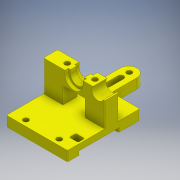
# Autodesk Inventor part: Extruder Mount
Saved by Autodesk Inventor 2016 (Build 200138000, 138)
## iProperties
Created: 2016-03-27
Part Number: Extruder Mount
Material: ABS Plastic
Document SubType Name: Modeling
Designer: Scott
Mass: 47.0424 g
Surface Area: 151.913 cm^2
Volume: 44.3796 cm^3
Density: 1.06 g/cm^3
Appearance: Smooth - Yellow
Author: Scott
Autodesk Inventor part; units mm, degrees
ref_plane "YZ Plane" through (0, 0, 0) normal (1, 0, 0) x (0, 1, 0)
ref_plane "XZ Plane" through (0, 0, 0) normal (0, 1, 0) x (-1, 0, 0)
sketch "Sketch1" plane through (0, 0, 0) normal (0, 0, 1) x (1, 0, 0)
  line L0 (0, 0) -> (85, 0)
  line L1 (85, 0) -> (85, 83.5)
  line L2 (85, 83.5) -> (0, 83.5)
  line L3 (0, 83.5) -> (0, 0)
  dimension "d0" = 85
  dimension "d1" = 83.5
  constraints: 8 end point, 2 parallel, 1 horizontal, 1 perpendicular
  measures "d0" distance of L1.end L2.end
  measures "d1" distance of L0.end L1.end
extrude "Extrusion1" add sketch "Sketch1" along normal blind 5
sketch "Sketch10" plane through (0, 0, 5) normal (0, 0, 1) x (1, 0, 0)
  line L0 (85, 0) -> (85, 83.5) projected
  line L1 (85, 83.5) -> (0, 83.5) projected
  line L2 (0, 83.5) -> (0, 0) projected
  circle A0 centre (15.5, 75) radius 2.25 projected
  circle A1 centre (15.5, 75) radius 4
  circle A2 centre (33.5, 75) radius 4
  circle A3 centre (51.5, 75) radius 4
  circle A4 centre (69.5, 75) radius 4
  circle A5 centre (33.5, 51) radius 2.25 projected
  line L3 (0, 0) -> (85, 0) projected
  circle A6 centre (33.5, 30) radius 4
  circle A7 centre (51.5, 30) radius 4
  circle A8 centre (33.5, 6) radius 4
  circle A9 centre (51.5, 6) radius 4
  line L4 (85, 0) -> (85, 83.5) projected
  line L5 (85, 83.5) -> (0, 83.5) projected
  line L6 (0, 83.5) -> (0, 0) projected
  line L7 (0, 0) -> (85, 0) projected
  circle A10 centre (15.5, 51) radius 2.25 projected
  circle A11 centre (15.5, 51) radius 4
  circle A12 centre (33.5, 51) radius 4
  circle A13 centre (51.5, 51) radius 4
  circle A14 centre (69.5, 51) radius 4
  circle A15 centre (37.75, 40.5) radius 1.5 projected
  circle A16 centre (47.25, 40.5) radius 1.5 projected
  circle A17 centre (37.75, 40.5) radius 2.75
  circle A18 centre (47.25, 40.5) radius 2.75
  dimension "d73" = 8
  dimension "d152" = 5.5
  constraints: 14 centre point, 12 equal radius, 5 coincident
  measures "d73" diameter of A1
  measures "d152" diameter of A17
extrude "Extrusion21" add sketch "Sketch10" along normal blind 4 contours L3 L2 L1 L0 | A0 | A1 | A2 | A3 | A4 | A5 | A6 | A7 | A8 | A9 | A10 | A11 | A12 | A13 | A14 | A15 | A16 | A17 | A18
sketch "Sketch24" plane through (0, 0, 9) normal (0, 0, 1) x (1, 0, 0)
  line L0 (9.5, 63.9289) -> (9.5, 2) projected
  line L1 (75.5, 2) -> (75.5, 63.9289) projected
  line L2 (75.5, 63.9289) -> (75.5, 2) projected
  line L3 (9.5, 46.85) -> (75.5, 46.85)
  line L4 (75.5, 46.85) -> (75.5, 34.15)
  line L5 (75.5, 34.15) -> (9.5, 34.15)
  line L6 (9.5, 34.15) -> (9.5, 46.85)
  line L7 (0, 0) -> (85, 0) projected
  point P0 (11.5, 0)
  point P1 (73.5, 0)
  dimension "d173" = 12.7
  dimension "d174" = 34.15
  constraints: 8 end point, 2 parallel, 2 point on line, 1 horizontal, 1 perpendicular
  measures "d173" distance between parallel lines of L5 L3
  measures "d174" distance between parallel lines of L7 L5
extrude "Extrusion22" add sketch "Sketch24" along normal blind 28
sketch "Sketch25" plane through (2, 83.5, 0) normal (0, 1, 0) x (1, 0, 0)
  line L0 (40.5, -12) -> (40.5, -37) construction
  line L1 (73.5, -37) -> (7.5, -37) construction
  line L2 (30.5, -9) -> (30.5, -24.2)
  line L3 (30.5, -24.2) -> (50.5, -24.2)
  line L4 (83, -9) -> (-2, -9) projected
  line L5 (50.5, -24.2) -> (50.5, -9)
  line L6 (50.5, -9) -> (30.5, -9)
  point P0 (-2, 0)
  point P1 (0, -9)
  dimension "d177" = 20
  dimension "d348" = 15.2
  constraints: 10 end point, 1 collinear, 1 midpoint, 1 perpendicular, 1 vertical
  measures "d177" distance of L2.end L3.end
  measures "d348" distance of L2.start L2.end
extrude "Extrusion23" cut sketch "Sketch25" against normal through all
sketch "Sketch26" plane through (9.5, 46.85, 37) normal (0, 1, 0) x (1, 0, 0)
  line L0 (66, 0) -> (0, 0) projected
  line L1 (43, 12.8) -> (23, 12.8) projected
  line L2 (33, 12.8) -> (33, 0) construction
  arc A0 (39.25, 3.25) -> (26.75, 3.25) centre (33, 3.25) ccw
  line L3 (39.25, 3.25) -> (39.25, 0)
  line L4 (26.75, 3.25) -> (26.75, 0)
  point P0 (-9.5, 37)
  point P1 (43, 9.8)
  dimension "d182" = 12.5
  dimension "d183" = 3.25
  constraints: 6 end point, 3 point on line, 2 perpendicular, 2 point on circle, 2 tangent, 1 centre point, 1 midpoint, 2 other
  measures "d182" diameter of A0
  measures "d183" distance from line of L0 A0.centre
extrude "Extrusion24" cut sketch "Sketch26" against normal through all
sketch "Sketch27" plane through (75.5, 46.85, 37) normal (0, 1, 0) x (1, 0, 0)
  arc A0 (-26.75, 3.25) -> (-39.25, 3.25) centre (-33, 3.25) ccw projected
  line L0 (-26.75, 3.25) -> (-26.75, 0) projected
  line L1 (-39.25, 0) -> (-39.25, 3.25) projected
  line L2 (-41.25, 0) -> (-41.25, 3.25)
  arc A1 (-24.75, 3.25) -> (-41.25, 3.25) centre (-33, 3.25) ccw
  line L3 (-24.75, 3.25) -> (-24.75, 0)
  line L4 (-66, 0) -> (-39.25, 0) projected
  line L5 (-41.25, 0) -> (-39.25, 0)
  line L6 (-26.75, 0) -> (-24.75, 0)
  line L7 (0, 0) -> (-26.75, 0) projected
  point P0 (-75.5, 37)
  dimension "d186" = 16.5
  constraints: 8 end point, 2 collinear, 2 point on circle, 1 centre point, 2 other
  measures "d186" distance of L3.start L2.end
extrude "Extrusion25" cut sketch "Sketch27" against normal blind 3.95
sketch "Sketch28" plane through (9.5, 34.15, 9) normal (0, -1, 0) x (1, 0, 0)
  arc A0 (24.75, 24.75) -> (41.25, 24.75) centre (33, 24.75) ccw projected
  line L0 (24.75, 28) -> (24.75, 24.75) projected
  line L1 (41.25, 24.75) -> (41.25, 28) projected
  line L2 (39.25, 28) -> (66, 28) projected
  line L3 (0, 28) -> (26.75, 28) projected
  line L4 (26.75, 24.75) -> (26.75, 28) projected
  arc A1 (26.75, 24.75) -> (39.25, 24.75) centre (33, 24.75) ccw projected
  line L5 (39.25, 28) -> (39.25, 24.75) projected
  point P0 (-9.5, -9)
extrude "Extrusion26" cut sketch "Sketch28" against normal blind 3.1
sketch "Sketch39" plane through (32.5, 46.85, 24.2) normal (0, 1, 0) x (1, 0, 0)
  line L0 (0, 0) -> (0, 15.2) projected
  circle A0 centre (0, 7.6) radius 1.25
  point P0 (-32.5, 24.2)
  dimension "d263" = 2.5
  constraints: 1 centre point, 1 midpoint
  measures "d263" diameter of A0
extrude "Extrusion35" cut sketch "Sketch39" against normal blind 4
fillet "Fillet23" radius 1 1 edges at (31.25, 42.85, 16.6)
sketch "Sketch40" plane through (32.5, 46.85, 24.2) normal (0, 1, 0) x (1, 0, 0)
  line L0 (20, 15.2) -> (20, 0) projected
  line L1 (24, 7.35) -> (33, 7.35)
  line L2 (34, 8.35) -> (34, 8.6)
  line L3 (34, 8.6) -> (23, 8.6)
  line L4 (23, 8.6) -> (23, 8.35)
  arc A0 (23, 8.35) -> (24, 7.35) centre (24, 8.35) ccw
  arc A1 (33, 7.35) -> (34, 8.35) centre (33, 8.35) ccw
  line L5 (20, 0) -> (0, 0) projected
  point P0 (-32.5, 24.2)
  point P1 (23, 7.35)
  dimension "d267" = 1.25
  dimension "d268" = 3
  dimension "d269" = 14
  dimension "d270" = 1
  dimension "d332" = 8.6
  constraints: 8 end point, 4 point on circle, 4 tangent, 2 centre point, 2 parallel, 2 point on line, 1 equal radius, 1 horizontal, 1 perpendicular
  measures "d267" distance of L3.end point (23, 7.35)
  measures "d268" distance between parallel lines of L4 L0
  measures "d269" distance between parallel lines of L2 L0
  measures "d270" radius of A0
  measures "d332" distance between parallel lines of L5 L3
revolve "Revolution1" cut sketch "Sketch40" angle 180 about axis through (66.5, 46.85, 15.6) along (1, 0, 0)
sketch "Sketch45" plane through (0, 0, 9) normal (0, 0, 1) x (1, 0, 0)
  line L0 (85, 83.5) -> (0, 83.5) projected
  line L1 (75.5, 46.85) -> (75.5, 63.9289) projected
  arc A0 (76.9645, 67.4645) -> (75.5, 63.9289) centre (80.5, 63.9289) ccw projected
  line L2 (76.9645, 67.4645) -> (84.4142, 74.9142) projected
  arc A1 (84.4142, 74.9142) -> (85, 76.3284) centre (83, 76.3284) ccw projected
  line L3 (85, 0) -> (85, 83.5) projected
  arc A2 (85, 81.5) -> (83, 83.5) centre (83, 81.5) ccw projected
  line L4 (85, 83.5) -> (0, 83.5) projected
  line L5 (75.5, 63.5) -> (85, 63.5)
  line L6 (85, 63.5) -> (85, 83.5)
  line L7 (85, 83.5) -> (75.5, 83.5)
  line L8 (75.5, 83.5) -> (75.5, 63.5)
  point P0 (0, 0)
  point P1 (43, 83.5)
  point P2 (75.5, 58.85)
  point P3 (41, 83.5)
  point P4 (75.5, 56.85)
  point P5 (2, 83.5)
  dimension "d301" = 20
  constraints: 9 end point, 2 parallel, 1 collinear, 1 horizontal, 1 perpendicular, 1 point on line
  measures "d301" distance between parallel lines of L0 L5
extrude "Extrusion39" cut sketch "Sketch45" against normal through all
sketch "Sketch51" plane through (0, 0, 0) normal (0, 0, -1) x (-1, 0, 0)
  line L0 (-75.5, 46.85) -> (-75.5, 34.15) construction
  line L1 (-9.5, 34.15) -> (-9.5, 46.85) construction
  line L2 (-75.5, 40.5) -> (-9.5, 40.5) construction
  line L3 (-75.5, 83.5) -> (0, 83.5) projected
  line L4 (0, 0) -> (-85, 0) projected
  line L5 (-70, 83.5) -> (-85, 83.5)
  line L6 (-85, 83.5) -> (-85, 0)
  line L7 (-85, 0) -> (-70, 0)
  line L8 (-70, 0) -> (-70, 83.5)
  line L9 (-42.5, 100.2) -> (-42.5, -16.7) projected
  line L10 (-15, 83.5) -> (0, 83.5)
  line L11 (0, 83.5) -> (0, 0)
  line L12 (0, 0) -> (-15, 0)
  line L13 (-15, 0) -> (-15, 83.5)
  dimension "d349" = 27.5
  dimension "d350" = 27.5
  constraints: 18 end point, 4 parallel, 2 horizontal, 2 midpoint, 2 perpendicular, 2 point on line
  measures "d349" distance between parallel lines of L8 L9
  measures "d350" distance between parallel lines of L13 L9
extrude "Extrusion43" cut sketch "Sketch51" against normal through all contours L3 L8 L4 L6 L5 | L3 L11 L4 L13
sketch "Sketch52" plane through (0, 0, 0) normal (0, 0, -1) x (-1, 0, 0)
  line L0 (-15, 46.85) -> (-15, 34.15) construction
  line L1 (-70, 34.15) -> (-70, 46.85) construction
  line L2 (-42.5, 100.2) -> (-42.5, -16.7) construction
  line L3 (-70, 83.5) -> (-15, 83.5) construction
  line L4 (-70, 83.5) -> (-70, 0) construction
  line L5 (-15, 0) -> (-70, 0) construction
  line L6 (-15, 0) -> (-15, 83.5) construction
  line L7 (-70, 83.5) -> (-15, 83.5) construction
  line L8 (-15, 83.5) -> (-15, 46.85) projected
  line L9 (-70, 83.5) -> (-15, 83.5)
  line L10 (-15, 83.5) -> (-15, 65.75)
  line L11 (-15, 65.75) -> (-70, 65.75)
  line L12 (-70, 65.75) -> (-70, 83.5)
  line L13 (-70, 41.75) -> (-15, 41.75) construction
  line L14 (-15, 0) -> (-70, 0) projected
  line L15 (-15, 34.15) -> (-15, 0) projected
  line L16 (-70, 0) -> (-15, 0)
  line L17 (-15, 0) -> (-15, 0.75)
  line L18 (-15, 0.75) -> (-70, 0.75)
  line L19 (-70, 0.75) -> (-70, 0)
  point P0 (0, 0)
  dimension "d353" = 24
  dimension "d373" = 65
  constraints: 18 end point, 4 parallel, 2 horizontal, 2 midpoint, 2 perpendicular, 2 point on line
  measures "d353" distance between parallel lines of L11 L13
  measures "d373" distance between parallel lines of L18 L11
extrude "Extrusion44" cut sketch "Sketch52" against normal through all
sketch "Sketch55" plane through (0, 0, 0) normal (0, 0, -1) x (-1, 0, 0)
  line L0 (-15, 0.75) -> (-15, 65.75) projected
  line L1 (-15, 65.75) -> (-15, 46.85) projected
  line L2 (-15, 34.15) -> (-15, 0.75) projected
  line L3 (-26, 46.75) -> (-15, 46.75)
  line L4 (-15, 46.75) -> (-15, 11.75)
  line L5 (-15, 11.75) -> (-26, 11.75)
  line L6 (-26, 11.75) -> (-26, 46.75)
  point P0 (0, 0)
  dimension "d374" = 19
  dimension "d375" = 11
  dimension "d376" = 11
  constraints: 8 end point, 2 parallel, 1 horizontal, 1 perpendicular, 1 point on line
  measures "d374" distance from line of L0.end L3
  measures "d375" distance from line of L0.start L5
  measures "d376" distance of L3.start L3.end
extrude "Extrusion45" cut sketch "Sketch55" against normal blind 3.5
sketch "Sketch56" plane through (0, 0, 0) normal (0, 0, -1) x (-1, 0, 0)
  line L0 (-70, 65.75) -> (-15, 65.75) construction
  line L1 (-42.5, 65.75) -> (-42.5, 0.75) construction
  line L2 (-15, 0.75) -> (-70, 0.75) construction
  line L3 (-54.5, 45.25) -> (-30.5, 45.25) construction
  line L4 (-30.5, 45.25) -> (-30.5, 21.25) construction
  line L5 (-30.5, 21.25) -> (-54.5, 21.25) construction
  line L6 (-54.5, 21.25) -> (-54.5, 45.25) construction
  line L7 (-30.5, 45.25) -> (-54.5, 21.25) construction
  line L8 (-54.5, 45.25) -> (-30.5, 21.25) construction
  point P0 (0, 0)
  point P1 (-42.5, 33.25)
  dimension "d379" = 24
  dimension "d380" = 24
  constraints: 14 end point, 4 midpoint, 3 coincident, 2 parallel, 1 horizontal, 1 perpendicular, 1 point on line
  measures "d379" distance of L3.start L3.end
  measures "d380" distance of L3.end L4.end
hole "Hole14" at (42.5, 33.25, 0) at (54.5, 45.25, 0) at (54.5, 21.25, 0) at (30.5, 21.25, 0) at (30.5, 45.25, 0) direction (0, 0, 1) diameter 3 depth 8
sketch "Sketch57" plane through (0, 0, 0) normal (0, 0, -1) x (-1, 0, 0)
  circle A0 centre (-42.5, 33.25) radius 1.5 projected
  point P0 (0, 0)
  constraints: 1 coincident
hole "Hole15" at (42.5, 33.25, 0) direction (0, 0, 1) diameter 4.7 depth 5
ref_plane "Work Plane14" through (42.5, 37.25, 33.75) normal (1, 0, 0) x (0, -1, 0)
sketch "Sketch58" plane through (0, 0, 3.5) normal (0, 0, -1) x (-1, 0, 0)
  circle A0 centre (-42.5, 33.25) radius 2.35 construction
  line L0 (-42.5, 33.25) -> (-7.5484, 33.25) construction
  line L1 (-15, 46.75) -> (-15, 11.75) construction
  line L2 (-26, 46.75) -> (-15, 46.75) construction
  line L3 (-26, 11.75) -> (-26, 46.75) construction
  line L4 (-15, 11.75) -> (-26, 11.75) construction
  line L5 (-25.2, 39.25) -> (-15.8, 39.25)
  line L6 (-15.8, 39.25) -> (-15.8, 27.25)
  line L7 (-15.8, 27.25) -> (-25.2, 27.25)
  line L8 (-25.2, 27.25) -> (-25.2, 39.25)
  point P0 (0, 0)
  dimension "d396" = 6
  dimension "d397" = 6
  dimension "d398" = 0.8
  dimension "d399" = 0.8
  constraints: 10 end point, 2 horizontal, 2 parallel, 1 perpendicular
  measures "d396" distance between parallel lines of L0 L5
  measures "d397" distance between parallel lines of L0 L7
  measures "d398" distance between parallel lines of L1 L6
  measures "d399" distance between parallel lines of L3 L8
extrude "Extrusion46" cut sketch "Sketch58" against normal blind 1.5
sketch "Sketch59" plane through (0, 0, 3.5) normal (0, 0, -1) x (-1, 0, 0)
  circle A0 centre (-42.5, 33.25) radius 2.35 construction
  line L0 (-42.5, 33.25) -> (-9.4661, 33.25) construction
  line L1 (-20.5, 50.9301) -> (-20.5, 7.336) construction
  line L2 (-15, 46.75) -> (-15, 11.75) projected
  point P0 (0, 0)
  point P1 (-20.5, 42.775)
  point P2 (-20.5, 23.725)
  dimension "d402" = 5.5
  dimension "d403" = 9.525
  dimension "d404" = 9.525
  constraints: 4 end point, 2 point on line, 1 horizontal, 1 vertical
  measures "d402" distance between parallel lines of L2 L1
  measures "d403" distance from line of L0 point (-20.5, 42.775)
  measures "d404" distance from line of L0 point (-20.5, 23.725)
hole "Hole16" at (20.5, 42.775, 3.5) at (20.5, 23.725, 3.5) direction (0, 0, 1) diameter 4.7 depth 5
sketch "Sketch60" plane through (32.5, 46.85, 24.2) normal (0, 1, 0) x (1, 0, 0)
  arc A0 (16.25, -9.55) -> (3.75, -9.55) centre (10, -9.55) ccw projected
  line L0 (37.5, -12.8) -> (37.5, 15.2) projected
  line L1 (10, -9.55) -> (43.533, -9.55) construction
  line L2 (37.5, -6.8) -> (36.2631, -6.8)
  line L3 (37.5, -12.8) -> (18.25, -12.8) projected
  arc A1 (36.2631, -6.8) -> (27.0629, -12.8) centre (31.5, -9.55) ccw
  point P0 (-32.5, 24.2)
  dimension "d412" = 6
  dimension "d414" = 5.5
  dimension "d415" = 6
  constraints: 4 end point, 3 point on line, 2 horizontal, 2 point on circle, 1 centre point
  measures "d412" distance from line of L0 A1.centre
  measures "d414" radius of A1
  measures "d415" distance between parallel lines of L3 L2
extrude "Extrusion47" cut sketch "Sketch60" against normal blind 20
mirror "Mirror6" about plane through (42.5, 37.25, 33.75) normal (1, 0, 0) of "Extrusion45", "Extrusion46", "Hole16"
sketch "Sketch62" plane through (42.5, 37.25, 33.75) normal (1, 0, 0) x (0, -1, 0)
  line L0 (-9.5, 33.75) -> (25.5, 33.75) projected
  line L1 (25.5, 33.75) -> (36.5, 33.75) projected
  line L2 (36.5, 33.75) -> (25.5, 33.75) projected
  line L3 (25.5, 33.75) -> (-9.5, 33.75) projected
  line L4 (-9.5, 33.75) -> (-28.5, 33.75) projected
  line L5 (-28.5, 33.75) -> (-9.5, 33.75) projected
  line L6 (-9.5, 33.75) -> (-6.5, 33.75) projected
  line L7 (14.5, 33.75) -> (17.5, 33.75) projected
  line L8 (-9.5, 33.75) -> (-6.5, 33.75) projected
  line L9 (14.5, 33.75) -> (17.5, 33.75) projected
  line L10 (1.65, 33.75) -> (6.35, 33.75) projected
  line L11 (36.5, 33.75) -> (36.5, 24.75) projected
  line L12 (36.5, 24.75) -> (36.5, 33.75) projected
  line L13 (-9.5, 30.25) -> (25.5, 30.25) construction
  line L14 (19.5, 31.25) -> (25.5, 31.25)
  line L15 (25.5, 31.25) -> (25.5, 28.25)
  line L16 (25.5, 28.25) -> (19.5, 28.25)
  line L17 (19.5, 28.25) -> (19.5, 31.25)
  point P0 (37.25, 33.75)
  dimension "d427" = 6
  dimension "d428" = 1
  dimension "d429" = 3
  dimension "d430" = 0
  constraints: 8 end point, 2 parallel, 1 horizontal, 1 perpendicular
  measures "d427" distance of L15.end L16.end
  measures "d428" distance between parallel lines of L13 L14
  measures "d429" distance of L14.end L15.end
  measures "d430" distance from line of L15 L13.end
extrude "Extrusion48" cut sketch "Sketch62" against normal blind 26
sketch "Sketch61" plane through (0, 0, 37) normal (0, 0, 1) x (1, 0, 0)
  line L0 (15, 46.85) -> (15, 34.15) projected
  line L1 (15, 40.5) -> (77.62, 40.5) construction
  line L2 (42.5, 78.9) -> (42.5, -13.15) construction
  point P0 (0, 0)
  point P1 (30, 40.5)
  point P2 (55, 40.5)
  dimension "d418" = 12.5
  dimension "d419" = 12.5
  constraints: 2 end point, 2 point on line, 1 horizontal, 1 midpoint
  measures "d418" distance from line of point (30, 40.5) L2
  measures "d419" distance from line of point (55, 40.5) L2
hole "Hole17" at (30, 40.5, 37) at (55, 40.5, 37) direction (0, 0, -1) diameter 3.5 depth 10 counterbore diameter 4.7 counterbore depth 5
mirror "Mirror7" about plane through (42.5, 37.25, 33.75) normal (1, 0, 0) of "Extrusion48"
sketch "Sketch63" plane through (0, 0, 9) normal (0, 0, 1) x (1, 0, 0)
  line L0 (16.5, 17.75) -> (68.5, 17.75) construction
  line L1 (68.5, 11.75) -> (68.5, 17.75) projected
  line L2 (16.5, 11.75) -> (68.5, 11.75) construction
  line L3 (59, 11.75) -> (70, 11.75) construction
  line L4 (68.5, 17.75) -> (60.5, 17.75)
  line L5 (60.5, 17.75) -> (60.5, 11.75)
  line L6 (60.5, 11.75) -> (68.5, 11.75)
  line L7 (68.5, 11.75) -> (68.5, 17.75)
  point P0 (0, 0)
  dimension "d433" = 8
  constraints: 8 end point, 2 parallel, 1 horizontal, 1 perpendicular, 1 point on line
  measures "d433" distance between parallel lines of L1 L5
extrude "Extrusion49" cut sketch "Sketch63" against normal through all
sketch "Sketch64" plane through (16.5, 11.75, 5.5) normal (0, 0, -1) x (-1, 0, 0)
  line L0 (-44, 6) -> (-44, 0) projected
  line L1 (0, 0) -> (-44, 0) projected
  line L2 (0, 0) -> (0, 6) projected
  line L3 (0, 6) -> (-44, 6) projected
  line L4 (-9.5, 6) -> (0, 6) projected
  line L5 (0, 0) -> (-44, 0) projected
  line L6 (0, 6) -> (-8, 6)
  line L7 (-8, 6) -> (-8, 0)
  line L8 (-8, 0) -> (0, 0)
  line L9 (0, 0) -> (0, 6)
  point P0 (16.5, -11.75)
  dimension "d436" = 8
  constraints: 8 end point, 2 parallel, 1 horizontal, 1 perpendicular, 1 point on line
  measures "d436" distance between parallel lines of L2 L7
extrude "Extrusion50" cut sketch "Sketch64" against normal blind 2 contours L7 L3 L2 L1
chamfer "Chamfer2" distance 2 angle 45 1 edges at (24.5, 14.75, 5.5)
fillet "Fillet30" radius 1 4 edges at (60.5, 17.75, 7.25) (60.5, 11.75, 7.25) (68.5, 11.75, 6.25) (68.5, 17.75, 6.25)
fillet "Fillet31" radius 1 12 edges at (70, 65.75, 4.5) (15, 65.75, 4.5) (15, 46.85, 23) (15, 34.15, 23) (15, 0.75, 4.5) (70, 0.75, 4.5) (70, 34.15, 20) (70, 46.85, 20) (70, 46.75, 1.75) (70, 11.75, 1.75) (15, 46.75, 1.75) (15, 11.75, 1.75)
sketch "Sketch65" plane through (0, 0, 0) normal (0, 0, -1) x (-1, 0, 0)
  line L0 (-69, 65.75) -> (-16, 65.75) projected
  line L1 (-44.5, 96.25) -> (-29.5, 96.25)
  line L2 (-29.5, 96.25) -> (-29.5, 65.75)
  line L3 (-29.5, 65.75) -> (-44.5, 65.75)
  line L4 (-44.5, 65.75) -> (-44.5, 96.25)
  line L5 (-15, 47.75) -> (-15, 64.75) projected
  point P0 (0, 0)
  dimension "d444" = 30.5
  dimension "d445" = 14.5
  dimension "d446" = 15
  constraints: 8 end point, 2 parallel, 1 horizontal, 1 perpendicular, 1 point on line
  measures "d444" distance of L1.end L2.end
  measures "d445" distance between parallel lines of L5 L2
  measures "d446" distance of L1.start L1.end
extrude "Extrusion51" add sketch "Sketch65" against normal up to surface (9 mm away)
sketch "Sketch66" plane through (0, 0, 9) normal (0, 0, 1) x (1, 0, 0)
  line L0 (32.5, 46.85) -> (32.5, 34.15) projected
  line L1 (16, 46.85) -> (32.5, 46.85) projected
  point P0 (0, 0)
  point P1 (37, 89.35)
  dimension "d449" = 4.5
  dimension "d450" = 42.5
  measures "d449" distance from line of point (37, 89.35) L0
  measures "d450" distance from line of L1 point (37, 89.35)
hole "Hole18" at (37, 89.35, 9) direction (0, 0, -1) diameter 3.5 depth 8 counterbore diameter 4.7 counterbore depth 5
fillet "Fillet32" radius 7.5 2 edges at (29.5, 96.25, 4.5) (44.5, 96.25, 4.5)
fillet "Fillet33" radius 2 2 edges at (44.5, 65.75, 4.5) (29.5, 65.75, 4.5)
sketch "Sketch67" plane through (0, 0, 9) normal (0, 0, 1) x (1, 0, 0)
  line L0 (37, 81.85) -> (37, 69.35) construction
  line L1 (34.5, 81.85) -> (34.5, 69.35)
  line L2 (39.5, 69.35) -> (39.5, 81.85)
  arc A0 (39.5, 81.85) -> (34.5, 81.85) centre (37, 81.85) ccw
  arc A1 (34.5, 69.35) -> (39.5, 69.35) centre (37, 69.35) ccw
  circle A2 centre (37, 89.35) radius 2.35 projected
  point P0 (0, 0)
  point P1 (37, 75.6)
  dimension "d460" = 7.5
  dimension "d461" = 12.5
  dimension "d462" = 0
  dimension "d463" = 2.5
  constraints: 8 end point, 4 point on circle, 4 tangent, 2 centre point, 1 midpoint, 1 parallel, 1 vertical
  measures "d460" distance of A2.centre L0.start
  measures "d461" distance of L0.start L0.end
  measures "d462" distance from line of A2.centre L0
  measures "d463" radius of A0
extrude "Extrusion52" cut sketch "Sketch67" against normal through all contours A0 L2 A1 L1
sketch "Sketch68" plane through (0, 0, 9) normal (0, 0, 1) x (1, 0, 0)
  line L0 (42.5, 115.5) -> (42.5, -19.25) projected
  line L1 (16, 0.75) -> (69, 0.75) projected
  point P0 (0, 0)
  point P1 (27.5, 5.75)
  point P2 (57.5, 5.75)
  dimension "d466" = 15
  dimension "d467" = 15
  dimension "d468" = 5
  dimension "d469" = 5
  measures "d466" distance from line of L0 point (57.5, 5.75)
  measures "d467" distance from line of L0 point (27.5, 5.75)
  measures "d468" distance from line of L1 point (57.5, 5.75)
  measures "d469" distance from line of point (27.5, 5.75) L1
hole "Hole19" at (27.5, 5.75, 9) at (57.5, 5.75, 9) direction (0, 0, -1) diameter 3.5 depth 8 counterbore diameter 4.7 counterbore depth 5
body "Solid1"
